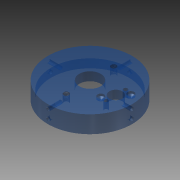
# Autodesk Inventor part: 13_1087_030
Saved by Autodesk Inventor 2014 SP1 (Build 180222100, 222)
## iProperties
Created: 2013-09-17
Part Number: 13_1087_030
Material: Allgemein
Document SubType Name: Modeling
Designer: vogel
Density: 1 g/cm^3
Appearance: Olivgrün
Author: vogel
Autodesk Inventor part; units mm, degrees
ref_plane "XZ Plane" through (0, 0, 0) normal (0, 1, 0) x (-1, 0, 0)
sketch "Skizze1" plane through (0, 0, 0) normal (0, 0, 1) x (1, 0, 0)
  line L0 (-44.1689, 0) -> (40.5177, 0) projected
  line L1 (0, -38.9628) -> (0, 40.9677) projected
  circle A0 centre (0, 0) radius 19.5
  dimension "d0" = 39
  constraints: 1 centre point, 1 coincident
  measures "d0" diameter of A0
extrude "Extrusion1" add sketch "Skizze1" along normal blind 4
hole "Bohrung1" at (0, 0, 4) direction (0, 0, -1) diameter 10 end through all
sketch "Skizze2" plane through (0, 0, 4) normal (0, 0, 1) x (1, 0, 0)
  circle A0 centre (0, 0) radius 5 projected
  line L0 (-44.1689, 0) -> (40.5177, 0) projected
  line L1 (0, -38.9628) -> (0, 40.9677) projected
  point P0 (12, 0)
  dimension "d14" = 12
  constraints: 1 point on line
  measures "d14" distance of point (12, 0) A0.centre
hole "Bohrung2" at (12, 0, 4) direction (0, 0, -1) diameter 6 end through all
sketch "Skizze5" plane through (0, 0, 4) normal (0, 0, 1) x (1, 0, 0)
  circle A0 centre (9, -4) radius 0.7 projected
  circle A1 centre (15, 4) radius 0.7 projected
  constraints: 2 coincident
hole "Bohrung4" at (9, -4, 4) at (15, 4, 4) direction (0, 0, -1) diameter 3 depth 1 tip angle 118
sketch "Skizze7" plane through (0, 0, 4) normal (0, 0, 1) x (1, 0, 0)
  line L0 (0, -38.9628) -> (0, 40.9677) projected
  line L1 (-44.1689, 0) -> (40.5177, 0) projected
  point P0 (12, -4.5)
  point P1 (12, 4.5)
  dimension "d39" = 12
  dimension "d40" = 9
  constraints: 1 symmetric about line
  measures "d39" distance from line of L0 point (12, -4.5)
  measures "d40" distance of point (12, 4.5) point (12, -4.5)
hole "Bohrung5" at (12, -4.5, 4) at (12, 4.5, 4) direction (0, 0, -1) diameter 1.8 end through all
sketch "Skizze9" plane through (0, 0, 0) normal (0, 0, -1) x (-1, 0, 0)
  circle A0 centre (0, 0) radius 19.5 projected
  circle A1 centre (0, 0) radius 18
  dimension "d58" = 1.5
  constraints: 1 centre point, 1 coincident
  measures "d58" radial gap between concentric circles of A0 A1
extrude "Extrusion3" add sketch "Skizze9" along normal blind 4
ref_plane "Arbeitsebene1" through (-19.5, 0, 0) normal (1, 0, 0) x (0, 1, 0)
sketch "Skizze10" plane through (-19.5, 0, 0) normal (1, 0, 0) x (0, 1, 0)
  line L0 (-5.4, 4) -> (-3.6, 4) projected
  line L1 (3.6, 4) -> (5.4, 4) projected
  line L2 (-19.5, 4) -> (19.5, 4) projected
  line L3 (-3, 4) -> (3, 4) projected
  line L4 (-5, 4) -> (5, 4) projected
  line L5 (19.5, 4) -> (-19.5, 4) projected
  line L6 (-34.9563, 0) -> (28.576, 0) projected
  line L7 (0, -5.6) -> (0, 5.6) projected
  point P0 (0, 0)
  point P1 (-5.5, 4)
  point P2 (-2.5, 4)
  point P3 (2.5, 4)
  point P4 (5.5, 4)
  point P5 (0, 2)
  point P6 (0, -2)
  dimension "d63" = 2
  dimension "d104" = 4
  constraints: 2 point on line
  measures "d63" distance from line of point (0, 2) L3
  measures "d104" distance of point (0, -2) point (0, 2)
hole "Bohrung7" at (-19.5, 0, 2) at (-19.5, 0, -2) direction (1, 0, 0) diameter 1.567 depth 6 tip angle 118 thread size "M2x0.4" class "6H" standard "ISO Metric profile"
sketch "Skizze11" plane through (0, 0, 4) normal (0, 0, 1) x (1, 0, 0)
  circle A0 centre (12, -4.5) radius 0.9 projected
  circle A1 centre (12, 4.5) radius 0.9 projected
  circle A2 centre (9, -4) radius 1.5 projected
  circle A3 centre (15, 4) radius 1.5 projected
  circle A4 centre (12, 0) radius 3 projected
  circle A5 centre (0, 0) radius 5 projected
  circle A6 centre (0, 0) radius 19.5 projected
  line L0 (0, 0) -> (-19.0596, 19.0596)
  line L1 (-27.3, 0) -> (27.3, 0) projected
  line L2 (0, -35.3992) -> (0, 31.2338) projected
  dimension "d71" = 45
  constraints: 2 end point, 1 coincident
  measures "d71" angle of L0 L1
ref_plane "Arbeitsebene4" through (13.7886, 13.7886, 0) normal (0.7071, 0.7071, 0) x (-0.7071, 0.7071, 0)
pattern_circular "Runde Anordnung1" count 4 over 360 about axis through (0, 0, 0) along (0, 0, 1) of "Bohrung7"
sketch "Skizze14" plane through (0, 0, 4) normal (0, 0, 1) x (1, 0, 0)
  line L0 (-27.3, 0) -> (27.3, 0) projected
  line L1 (0, -35.3992) -> (0, 31.2338) projected
  point P0 (0, 11)
  point P1 (0, -11)
  dimension "d96" = 22
  constraints: 2 point on line, 1 symmetric about line
  measures "d96" distance of point (0, -11) point (0, 11)
hole "Bohrung10" at (0, 11, 4) at (0, -11, 4) direction (0, 0, -1) diameter 2.459 end through all thread size "M3x0.5" class "6H" standard "ISO Metric profile"
